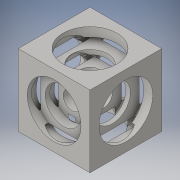
# Autodesk Inventor part: turners cube
Saved by Autodesk Inventor 2016 (Build 200138000, 138)
## iProperties
Created: 2017-02-22
Part Number: turners cube
Material: Generic
Document SubType Name: Modeling
Designer: jwillauer
Density: 1 g/cm^3
Appearance: Default
Author: jwillauer
Autodesk Inventor part; units mm, degrees
ref_plane "YZ Plane" through (0, 0, 0) normal (1, 0, 0) x (0, 1, 0)
ref_plane "XZ Plane" through (0, 0, 0) normal (0, 1, 0) x (-1, 0, 0)
ref_plane "XY Plane" through (0, 0, 0) normal (0, 0, 1) x (1, 0, 0)
sketch "Sketch1" plane through (0, 0, 0) normal (0, 0, 1) x (1, 0, 0)
  line L0 (-16.3593, 7.4143) -> (9.0407, 7.4143)
  line L1 (9.0407, 7.4143) -> (9.0407, -17.9857)
  line L2 (9.0407, -17.9857) -> (-16.3593, -17.9857)
  line L3 (-16.3593, -17.9857) -> (-16.3593, 7.4143)
  point P0 (0, 0)
  dimension "d0" = 25.4
  dimension "d1" = 25.4
  constraints: 8 end point, 2 parallel, 1 horizontal, 1 perpendicular
  measures "d0" distance of L0.start L0.end
  measures "d1" distance of L2.end L0.start
extrude "Extrusion1" add sketch "Sketch1" along normal blind 25.4
sketch "Sketch8" plane through (-16.3593, -17.9857, 0) normal (-1, 0, 0) x (0, 0, 1)
  line L0 (9.525, 15.875) -> (12.7, 12.7) projected
  circle A0 centre (12.7, 12.7) radius 3.175
  point P0 (0, 17.9857)
  dimension "d26" = 6.35
  constraints: 1 centre point
  measures "d26" diameter of A0
extrude "Extrusion8" cut sketch "Sketch8" against normal through all
sketch "Sketch11" plane through (0, 0, 25.4) normal (0, 0, 1) x (1, 0, 0)
  circle A0 centre (-3.6593, -5.2857) radius 3.175
  line L0 (-16.3593, -17.9857) -> (9.0407, -17.9857) projected
  line L1 (9.0407, -17.9857) -> (9.0407, 7.4143) projected
  point P0 (0, 0)
  dimension "d33" = 6.35
  dimension "d34" = 12.7
  dimension "d35" = 12.7
  constraints: 1 centre point
  measures "d33" diameter of A0
  measures "d34" distance from line of L0 A0.centre
  measures "d35" distance from line of L1 A0.centre
extrude "Extrusion11" cut sketch "Sketch11" against normal through all
sketch "Sketch12" plane through (-16.3593, 7.4143, 0) normal (0, 1, 0) x (1, 0, 0)
  line L0 (12.7, -12.7) -> (9.525, -9.525) projected
  circle A0 centre (12.7, -12.7) radius 3.175
  point P0 (16.3593, 0)
  dimension "d38" = 6.35
  constraints: 1 centre point
  measures "d38" diameter of A0
extrude "Extrusion12" cut sketch "Sketch12" against normal through all
sketch "Sketch13" plane through (0, 0, 0) normal (0, 0, -1) x (-1, 0, 0)
  circle A0 centre (3.6593, -5.2857) radius 6.35
  circle A1 centre (3.6593, -5.2857) radius 3.175 projected
  point P0 (0, 0)
  dimension "d41" = 12.7
  constraints: 1 centre point, 1 concentric
  measures "d41" diameter of A0
extrude "Extrusion13" cut sketch "Sketch13" against normal blind 6.35
sketch "Sketch14" plane through (0, 0, 25.4) normal (0, 0, 1) x (1, 0, 0)
  circle A0 centre (-3.6593, -5.2857) radius 6.35
  circle A1 centre (-3.6593, -5.2857) radius 3.175 projected
  point P0 (0, 0)
  dimension "d44" = 12.7
  constraints: 1 centre point, 1 concentric
  measures "d44" diameter of A0
extrude "Extrusion14" cut sketch "Sketch14" against normal blind 6.35
sketch "Sketch15" plane through (-16.3593, 7.4143, 0) normal (0, 1, 0) x (1, 0, 0)
  circle A0 centre (12.7, -12.7) radius 6.35
  circle A1 centre (12.7, -12.7) radius 3.175 projected
  point P0 (16.3593, 0)
  dimension "d47" = 12.7
  constraints: 1 centre point, 1 concentric
  measures "d47" diameter of A0
extrude "Extrusion15" cut sketch "Sketch15" against normal blind 6.35
sketch "Sketch16" plane through (9.0407, -17.9857, 0) normal (1, 0, 0) x (0, 0, -1)
  circle A0 centre (-12.7, 12.7) radius 6.35
  circle A1 centre (-12.7, 12.7) radius 3.175 projected
  point P0 (0, 17.9857)
  dimension "d50" = 12.7
  constraints: 1 centre point, 1 concentric
  measures "d50" diameter of A0
extrude "Extrusion16" cut sketch "Sketch16" against normal blind 6.35
sketch "Sketch17" plane through (-16.3593, -17.9857, 0) normal (0, -1, 0) x (1, 0, 0)
  circle A0 centre (12.7, 12.7) radius 6.35
  circle A1 centre (12.7, 12.7) radius 3.175 projected
  point P0 (16.3593, 0)
  dimension "d53" = 12.7
  constraints: 1 centre point, 1 concentric
  measures "d53" diameter of A0
extrude "Extrusion17" cut sketch "Sketch17" against normal blind 6.35
sketch "Sketch18" plane through (-16.3593, -17.9857, 0) normal (-1, 0, 0) x (0, 0, 1)
  circle A0 centre (12.7, 12.7) radius 6.35
  circle A1 centre (12.7, 12.7) radius 3.175 projected
  point P0 (0, 17.9857)
  dimension "d56" = 12.7
  constraints: 1 centre point, 1 concentric
  measures "d56" diameter of A0
extrude "Extrusion18" cut sketch "Sketch18" against normal blind 6.35
sketch "Sketch19" plane through (9.0407, -17.9857, 0) normal (1, 0, 0) x (0, 0, -1)
  circle A0 centre (-12.7, 12.7) radius 9.525
  circle A1 centre (-12.7, 12.7) radius 6.35 projected
  point P0 (0, 17.9857)
  dimension "d59" = 19.05
  constraints: 1 centre point, 1 concentric
  measures "d59" diameter of A0
extrude "Extrusion19" cut sketch "Sketch19" against normal blind 3.175
sketch "Sketch20" plane through (0, 0, 25.4) normal (0, 0, 1) x (1, 0, 0)
  circle A0 centre (-3.6593, -5.2857) radius 9.525
  circle A1 centre (-3.6593, -5.2857) radius 6.35 projected
  point P0 (0, 0)
  dimension "d62" = 19.05
  constraints: 1 centre point, 1 concentric
  measures "d62" diameter of A0
extrude "Extrusion20" cut sketch "Sketch20" against normal blind 3.175
sketch "Sketch21" plane through (-16.3593, 7.4143, 0) normal (0, 1, 0) x (1, 0, 0)
  circle A0 centre (12.7, -12.7) radius 9.525
  circle A1 centre (12.7, -12.7) radius 6.35 projected
  point P0 (16.3593, 0)
  dimension "d65" = 19.05
  constraints: 1 centre point, 1 concentric
  measures "d65" diameter of A0
extrude "Extrusion21" cut sketch "Sketch21" against normal blind 3.175
sketch "Sketch22" plane through (-16.3593, -17.9857, 0) normal (0, -1, 0) x (1, 0, 0)
  circle A0 centre (12.7, 12.7) radius 9.525
  circle A1 centre (12.7, 12.7) radius 6.35 projected
  point P0 (16.3593, 0)
  dimension "d68" = 19.05
  constraints: 1 centre point, 1 concentric
  measures "d68" diameter of A0
extrude "Extrusion22" cut sketch "Sketch22" against normal blind 3.175
sketch "Sketch23" plane through (0, 0, 0) normal (0, 0, -1) x (-1, 0, 0)
  circle A0 centre (3.6593, -5.2857) radius 9.525
  circle A1 centre (3.6593, -5.2857) radius 6.35 projected
  point P0 (0, 0)
  dimension "d71" = 19.05
  constraints: 1 centre point, 1 concentric
  measures "d71" diameter of A0
extrude "Extrusion23" cut sketch "Sketch23" against normal blind 3.175
sketch "Sketch24" plane through (-16.3593, -17.9857, 0) normal (-1, 0, 0) x (0, 0, 1)
  circle A0 centre (12.7, 12.7) radius 9.525
  circle A1 centre (12.7, 12.7) radius 6.35 projected
  point P0 (0, 17.9857)
  dimension "d74" = 19.05
  constraints: 1 centre point, 1 concentric
  measures "d74" diameter of A0
extrude "Extrusion24" cut sketch "Sketch24" against normal blind 3.175
sketch "Sketch25" plane through (-10.0093, -17.9857, 0) normal (-1, 0, 0) x (0, 0, 1)
  circle A0 centre (12.804, 12.6209) radius 7.8204
  point P0 (0, 17.9857)
  constraints: 1 centre point
extrude "Extrusion25" cut sketch "Sketch25" against normal blind 1.5875
sketch "Sketch26" plane through (-13.1843, -17.9857, 0) normal (-1, 0, 0) x (0, 0, 1)
  circle A0 centre (12.7615, 12.6988) radius 11.2231
  point P0 (0, 17.9857)
  constraints: 1 centre point
extrude "Extrusion26" cut sketch "Sketch26" against normal blind 1.5875
sketch "Sketch27" plane through (-16.3593, 1.0643, 0) normal (0, 1, 0) x (1, 0, 0)
  circle A0 centre (12.9411, -12.8527) radius 8.8917
  point P0 (16.3593, 0)
  constraints: 1 centre point
extrude "Extrusion27" cut sketch "Sketch27" against normal blind 1.5875
sketch "Sketch28" plane through (-16.3593, 4.2393, 0) normal (0, 1, 0) x (1, 0, 0)
  circle A0 centre (12.7132, -12.8071) radius 12.1242
  point P0 (16.3593, 0)
  constraints: 1 centre point
extrude "Extrusion28" cut sketch "Sketch28" against normal blind 1.5875
sketch "Sketch29" plane through (2.6907, -17.9857, 0) normal (1, 0, 0) x (0, 0, -1)
  circle A0 centre (-12.7159, 12.6076) radius 7.7855
  point P0 (0, 17.9857)
  constraints: 1 centre point
extrude "Extrusion29" cut sketch "Sketch29" against normal blind 1.5875
sketch "Sketch30" plane through (5.8657, -17.9857, 0) normal (1, 0, 0) x (0, 0, -1)
  circle A0 centre (-12.7615, 12.7443) radius 11.2232
  point P0 (0, 17.9857)
  constraints: 1 centre point
extrude "Extrusion30" cut sketch "Sketch30" against normal blind 1.5875
sketch "Sketch31" plane through (-16.3593, -11.6357, 0) normal (0, -1, 0) x (1, 0, 0)
  circle A0 centre (12.6375, 12.7679) radius 6.4179
  line L0 (12.7, 6.35) -> (7.9375, 6.35) projected
  point P0 (16.3593, 0)
  constraints: 1 centre point, 1 tangent
extrude "Extrusion31" cut sketch "Sketch31" against normal blind 1.5875
sketch "Sketch32" plane through (-16.3593, -14.8107, 0) normal (0, -1, 0) x (1, 0, 0)
  arc A0 (0.5894, 12.7) -> (12.7, 0.6829) centre (12.7132, 12.8071) ccw projected
  circle A1 centre (12.4824, 12.6128) radius 11.9319
  point P0 (16.3593, 0)
  constraints: 3 other
extrude "Extrusion32" cut sketch "Sketch32" against normal blind 1.5875
body "Solid1"
